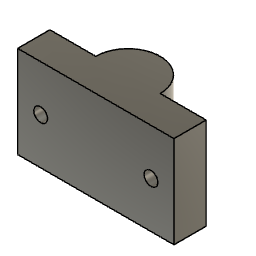
End_p (Autodesk Fusion 360 design; units mm, degrees)
Autodesk Fusion 360 part; units mm, degrees
sketch "Sketch1" plane through (0, 0, 0) normal (0, 0, 1) x (1, 0, 0)
  circle A0 centre (0, 0) radius 4
  circle A1 centre (0, 0) radius 7
  line L0 (0, -6) -> (0, -7.3)
  line L1 (0, -7) -> (17, -7)
  line L2 (17, -7) -> (17, 0)
  line L3 (17, 0) -> (0, 0)
  line L4 (0, 0) -> (0, -7)
  line L5 (0, -7) -> (-17, -7)
  line L6 (-17, -7) -> (-17, 0)
  line L7 (-17, 0) -> (0, 0)
  line L8 (0, 0) -> (0, -7)
  line L9 (0.2459, 6.9957) -> (17, 0)
  line L10 (0.2459, 6.9957) -> (-17, 0)
  dimension "d1" = 8
  dimension "d2" = 14
  dimension "d3" = 17
  dimension "d4" = 7
  constraint coincident A0.centre A1.centre
  constraint concentric A0 A1
  constraint vertical L0
  constraint horizontal L1
  constraint vertical L2
  constraint horizontal L3
  constraint vertical L4
  constraint coincident L0 L1.start
  constraint coincident A1 L1.start
  constraint symmetric L1.start L4 L5.start
  constraint symmetric L1.end L4 L5.end
  constraint symmetric L2.end L4 L6.end
  constraint symmetric A0.centre L4 A1.centre
  constraint coincident A1 L9.start
  measures "d1" diameter of A0
  measures "d2" diameter of A1
  measures "d3" distance of L1.start L1.end
  measures "d4" distance of L1.start A0.centre
extrude "Extrude1" add sketch "Sketch1" along normal blind 20 contours A0 A1 L0 L3 L4 L8 | A0 A1 L3 L7 L9 L10 | A0 A1 L0 L4 L7 L8 | A1 L1 L2 L3 | A1 L5 L6 L7 | A1 L9 | A1 L10
sketch "Sketch2" plane through (0, 0, 20) normal (0, 0, 1) x (-1, 0, 0)
  circle A0 centre (0, 0) radius 4
  line L0 (17, 7) -> (-17, 7)
  line L1 (-17, 7) -> (-17, 0)
  line L2 (-17, 0) -> (-7, 0)
  arc A1 (-7, 0) -> (7, 0) centre (0, 0) ccw
  line L3 (7, 0) -> (17, 0)
  line L4 (17, 0) -> (17, 7)
  circle A2 centre (0, 0) radius 4
  constraint concentric A0 A2
extrude "Extrude2" add sketch "Sketch2" against normal blind 10 contours A0 A2
sketch "Sketch3" plane through (0, 0, 0) normal (0, 1, 0) x (-1, 0, 0)
  line L0 (-17, 0) -> (-7, 0)
  line L1 (-7, 0) -> (-7, 20)
  line L2 (-7, 20) -> (-17, 20)
  line L3 (-17, 20) -> (-17, 0)
  line L4 (-12, 0) -> (-12, 20) construction
  line L5 (-17, 10) -> (-7, 10) construction
  circle A0 centre (-12, 10) radius 1.5
  line L6 (0, 20) -> (0, 0) construction
  circle A1 centre (12, 10) radius 1.5
  dimension "d9" = 3
  constraint midpoint L0 L4.start
  constraint midpoint L2 L4.end
  constraint midpoint L3 L5.start
  constraint midpoint L1 L5.end
  constraint midpoint L4 A0.centre
  constraint coincident L6.end origin
  constraint vertical L6
  constraint symmetric A0 L6 A1
  measures "d9" diameter of A0
hole "Hole1" at (12, 0, 10) at (-12, 0, 10) direction (0, -1, 0) diameter 3 depth 11 tip angle 118
